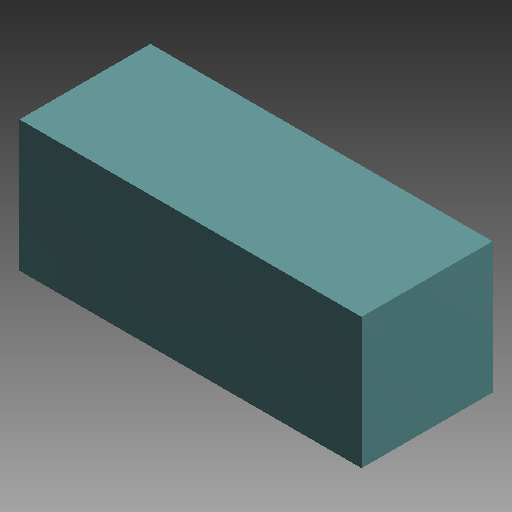
# Autodesk Inventor part: BLM41PG600SN1L
Saved by Autodesk Inventor 2018.2 (Build 222227000, 227)
## iProperties
Part Number: BLM41PG600SN1L
Material: Generic
Document SubType Name: Modeling
Designer: autocad
Appearance: L1806, BLM41PG600SN1L
Author: autocad
Autodesk Inventor part; units mm, degrees
ref_plane "YZ Plane" through (0, 0, 0) normal (1, 0, 0) x (0, 1, 0)
ref_plane "XZ Plane" through (0, 0, 0) normal (0, 1, 0) x (-1, 0, 0)
ref_plane "XY Plane" through (0, 0, 0) normal (0, 0, 1) x (1, 0, 0)
sketch "L1806, BLM41PG600SN1L_79" plane through (0, 0, 0) normal (0, 0, 1) x (1, 0, 0)
  line L0 (-2.35, 0.9) -> (2.35, 0.9)
  line L1 (2.35, 0.9) -> (2.35, -0.9)
  line L2 (2.35, -0.9) -> (-2.35, -0.9)
  line L3 (-2.35, -0.9) -> (-2.35, 0.9)
  constraints: 8 end point
extrude "Extrusion1" add sketch "L1806, BLM41PG600SN1L_79" along normal blind 1.8
body "Solid1"
